Autodesk Fusion 360 part; units mm, degrees
(part 2 of 25)
  arc A218 (53.5347, 54.332) -> (53.2751, 54.0724) centre (53.5347, 54.0724) ccw
  arc A219 (53.5347, 54.3066) -> (53.5347, 54.3574) centre (53.5347, 54.332) ccw
  arc A220 (53.5996, 53.1763) -> (53.5996, 53.1255) centre (53.5996, 53.1509) ccw
  arc A221 (53.8988, 54.0724) -> (53.9496, 54.0724) centre (53.9242, 54.0724) ccw
  arc A222 (52.7304, 52.8264) -> (52.7812, 52.8264) centre (52.7558, 52.8264) ccw
  arc A223 (53.9242, 54.0724) -> (53.6646, 54.332) centre (53.6646, 54.0724) ccw
  arc A224 (53.8988, 53.6829) -> (53.9496, 53.6829) centre (53.9242, 53.6829) ccw
  arc A225 (52.7558, 53.7083) -> (52.7558, 53.6575) centre (52.7558, 53.6829) ccw
  arc A226 (34.8662, 27.9667) -> (34.8822, 28.0149) centre (34.8742, 27.9908) ccw
  arc A227 (53.2497, 53.6829) -> (53.3005, 53.6829) centre (53.2751, 53.6829) ccw
  arc A228 (53.3005, 54.0724) -> (53.2497, 54.0724) centre (53.2751, 54.0724) ccw
  arc A229 (53.0804, 53.1255) -> (53.0804, 53.1763) centre (53.0804, 53.1509) ccw
  arc A230 (53.2751, 53.6575) -> (53.2751, 53.7083) centre (53.2751, 53.6829) ccw
  arc A231 (52.7812, 54.332) -> (52.7304, 54.332) centre (52.7558, 54.332) ccw
  arc A232 (56.4642, 52.4764) -> (56.4642, 52.5272) centre (56.4642, 52.5018) ccw
  arc A233 (51.1246, 29.8986) -> (51.1246, 29.9494) centre (51.1246, 29.924) ccw
  line L54 (29.7942, 28.6399) -> (29.7942, 28.2504)
  arc A234 (52.7812, 52.8264) -> (52.7304, 52.8264) centre (52.7558, 52.8264) ccw
  arc A235 (53.8988, 52.5018) -> (53.9496, 52.5018) centre (53.9242, 52.5018) ccw
  line L55 (53.9242, 52.8264) -> (53.9242, 52.5018)
  arc A236 (53.2497, 54.0724) -> (53.3005, 54.0724) centre (53.2751, 54.0724) ccw
  arc A237 (54.9481, 2.4638) -> (54.9481, 2.5146) centre (54.9481, 2.4892) ccw
  arc A238 (55.3212, 52.8264) -> (55.2704, 52.8264) centre (55.2958, 52.8264) ccw
  arc A239 (53.0804, 53.1763) -> (53.0804, 53.1255) centre (53.0804, 53.1509) ccw
  arc A240 (55.2958, 52.5272) -> (55.2958, 52.4764) centre (55.2958, 52.5018) ccw
  arc A241 (53.6646, 54.3574) -> (53.6646, 54.3066) centre (53.6646, 54.332) ccw
  arc A242 (55.6204, 53.1509) -> (55.2958, 52.8264) centre (55.6204, 52.8263) ccw
  arc A243 (55.2704, 52.8264) -> (55.3212, 52.8264) centre (55.2958, 52.8264) ccw
  arc A244 (52.7304, 52.5018) -> (52.7812, 52.5018) centre (52.7558, 52.5018) ccw
  arc A245 (53.8988, 52.8264) -> (53.9496, 52.8264) centre (53.9242, 52.8264) ccw
  arc A246 (53.9496, 54.0724) -> (53.8988, 54.0724) centre (53.9242, 54.0724) ccw
  line L56 (52.7558, 53.6829) -> (52.7558, 54.332)
  arc A247 (52.7304, 53.6829) -> (52.7812, 53.6829) centre (52.7558, 53.6829) ccw
  arc A248 (52.7558, 52.5272) -> (52.7558, 52.4764) centre (52.7558, 52.5018) ccw
  arc A249 (28.8854, 28.0162) -> (28.8854, 27.9654) centre (28.8854, 27.9908) ccw
  arc A250 (26.0778, 30.3771) -> (26.0938, 30.3289) centre (26.0858, 30.353) ccw
  line L57 (53.0804, 53.1509) -> (53.5996, 53.1509)
  arc A251 (26.0604, 29.2749) -> (26.1112, 29.2749) centre (26.0858, 29.2749) ccw
  arc A252 (33.7138, 28.4044) -> (33.6978, 28.3562) centre (33.7058, 28.3803) ccw
  arc A253 (53.9242, 52.8264) -> (53.5996, 53.1509) centre (53.5996, 52.8263) ccw
  line L58 (53.9242, 53.6829) -> (53.9242, 54.0724)
  line L59 (53.2751, 54.0724) -> (53.2751, 53.6829)
  arc A254 (29.8196, 28.6399) -> (29.7688, 28.6399) centre (29.7942, 28.6399) ccw
  line L60 (53.2751, 53.6829) -> (52.7558, 53.6829)
  line L61 (55.6204, 53.1509) -> (56.1396, 53.1509)
  line L62 (55.2958, 52.5018) -> (55.2958, 52.8264)
  arc A255 (56.1396, 53.1255) -> (56.1396, 53.1763) centre (56.1396, 53.1509) ccw
  arc A256 (61.5442, 52.8264) -> (61.2196, 53.1509) centre (61.2196, 52.8263) ccw
  arc A257 (56.23, 54.332) -> (56.1792, 54.332) centre (56.2046, 54.332) ccw
  arc A258 (58.1604, 53.1763) -> (58.1604, 53.1255) centre (58.1604, 53.1509) ccw
  line L63 (59.0042, 53.6829) -> (59.0042, 54.0075)
  arc A259 (59.0042, 54.0075) -> (58.3551, 54.0075) centre (58.6797, 54.0075) ccw
  arc A260 (55.3028, 53.967) -> (55.2888, 53.9181) centre (55.2958, 53.9426) ccw
  arc A261 (58.1604, 53.1509) -> (57.8358, 52.8264) centre (58.1604, 52.8263) ccw
  line L64 (56.2046, 53.6829) -> (56.2046, 54.332)
  arc A262 (58.3297, 54.0075) -> (58.3805, 54.0075) centre (58.3551, 54.0075) ccw
  arc A263 (57.8612, 52.8264) -> (57.8104, 52.8264) centre (57.8358, 52.8264) ccw
  arc A264 (57.8104, 53.6829) -> (57.8612, 53.6829) centre (57.8358, 53.6829) ccw
  arc A265 (56.1792, 53.6829) -> (56.23, 53.6829) centre (56.2046, 53.6829) ccw
  arc A266 (58.1604, 53.1255) -> (58.1604, 53.1763) centre (58.1604, 53.1509) ccw
  arc A267 (58.3551, 54.0724) -> (57.8358, 54.0724) centre (58.0954, 54.0724) ccw
  arc A268 (56.4896, 52.8264) -> (56.4388, 52.8264) centre (56.4642, 52.8264) ccw
  arc A269 (58.3297, 54.0724) -> (58.3805, 54.0724) centre (58.3551, 54.0724) ccw
  arc A270 (59.0296, 52.8264) -> (58.9788, 52.8264) centre (59.0042, 52.8264) ccw
  arc A271 (60.3758, 52.5272) -> (60.3758, 52.4764) centre (60.3758, 52.5018) ccw
  arc A272 (61.5442, 52.4764) -> (61.5442, 52.5272) centre (61.5442, 52.5018) ccw
  line L65 (61.5442, 52.5018) -> (60.3758, 52.5018)
  arc A273 (58.3297, 53.8127) -> (58.3805, 53.8127) centre (58.3551, 53.8127) ccw
  arc A274 (60.4012, 52.8264) -> (60.3504, 52.8264) centre (60.3758, 52.8264) ccw
  line L66 (59.0042, 52.5018) -> (57.8358, 52.5018)
  line L67 (55.9449, 54.1373) -> (56.4642, 54.1373)
  line L68 (59.0042, 52.8264) -> (59.0042, 52.5018)
  arc A275 (58.9788, 53.6829) -> (59.0296, 53.6829) centre (59.0042, 53.6829) ccw
  arc A276 (60.7004, 53.1509) -> (60.3758, 52.8264) centre (60.7004, 52.8263) ccw
  arc A277 (57.8104, 52.5018) -> (57.8612, 52.5018) centre (57.8358, 52.5018) ccw
  line L69 (60.7004, 53.1509) -> (61.2196, 53.1509)
  arc A278 (59.0042, 52.8264) -> (58.6796, 53.1509) centre (58.6796, 52.8263) ccw
  arc A279 (58.9788, 52.8264) -> (59.0296, 52.8264) centre (59.0042, 52.8264) ccw
  arc A280 (60.3504, 52.8264) -> (60.4012, 52.8264) centre (60.3758, 52.8264) ccw
  arc A281 (57.8612, 54.0724) -> (57.8104, 54.0724) centre (57.8358, 54.0724) ccw
  arc A282 (60.7004, 53.1763) -> (60.7004, 53.1255) centre (60.7004, 53.1509) ccw
  arc A283 (55.9449, 54.1627) -> (55.9449, 54.1119) centre (55.9449, 54.1373) ccw
  line L70 (57.8358, 52.5018) -> (57.8358, 52.8264)
  arc A284 (57.8104, 52.8264) -> (57.8612, 52.8264) centre (57.8358, 52.8264) ccw
  arc A285 (60.7004, 53.1255) -> (60.7004, 53.1763) centre (60.7004, 53.1509) ccw
  line L71 (58.3551, 54.0724) -> (58.3551, 53.8127)
  arc A286 (55.6204, 53.1763) -> (55.6204, 53.1255) centre (55.6204, 53.1509) ccw
  arc A287 (57.8358, 52.5272) -> (57.8358, 52.4764) centre (57.8358, 52.5018) ccw
  arc A288 (59.0042, 52.4764) -> (59.0042, 52.5272) centre (59.0042, 52.5018) ccw
  arc A289 (56.4642, 52.8264) -> (56.1396, 53.1509) centre (56.1396, 52.8263) ccw
  arc A290 (58.9788, 54.0075) -> (59.0296, 54.0075) centre (59.0042, 54.0075) ccw
  arc A291 (56.4388, 52.5018) -> (56.4896, 52.5018) centre (56.4642, 52.5018) ccw
  line L72 (56.4642, 52.8264) -> (56.4642, 52.5018)
  arc A292 (56.1976, 53.6585) -> (56.2115, 53.7073) centre (56.2045, 53.6829) ccw
  arc A293 (56.4642, 54.1119) -> (56.4642, 54.1627) centre (56.4642, 54.1373) ccw
  arc A294 (58.6796, 53.1255) -> (58.6796, 53.1763) centre (58.6796, 53.1509) ccw
  arc A295 (58.6796, 53.1763) -> (58.6796, 53.1255) centre (58.6796, 53.1509) ccw
  arc A296 (59.0296, 54.0075) -> (58.9788, 54.0075) centre (59.0042, 54.0075) ccw
  line L73 (58.1604, 53.1509) -> (58.6796, 53.1509)
  arc A297 (58.9788, 52.5018) -> (59.0296, 52.5018) centre (59.0042, 52.5018) ccw
  line L74 (55.2958, 53.9425) -> (56.2046, 53.6829)
  arc A298 (58.3805, 54.0724) -> (58.3297, 54.0724) centre (58.3551, 54.0724) ccw
  line L75 (57.8358, 53.6829) -> (57.8358, 54.0724)
  arc A299 (56.1396, 53.1763) -> (56.1396, 53.1255) centre (56.1396, 53.1509) ccw
  line L76 (60.3758, 52.5018) -> (60.3758, 52.8264)
  arc A300 (57.8104, 54.0724) -> (57.8612, 54.0724) centre (57.8358, 54.0724) ccw
  arc A301 (60.3504, 52.5018) -> (60.4012, 52.5018) centre (60.3758, 52.5018) ccw
  arc A302 (61.2196, 53.1255) -> (61.2196, 53.1763) centre (61.2196, 53.1509) ccw
  arc A303 (31.1578, 28.4044) -> (31.1738, 28.3562) centre (31.1658, 28.3803) ccw
  arc A304 (32.3422, 28.7456) -> (32.3262, 28.7938) centre (32.3342, 28.7697) ccw
  arc A305 (32.3262, 27.9667) -> (32.3422, 28.0149) centre (32.3342, 27.9908) ccw
  arc A306 (31.1738, 28.4044) -> (31.1578, 28.3562) centre (31.1658, 28.3803) ccw
  line L77 (31.4254, 29.1987) -> (31.1658, 29.5233)
  line L78 (61.5442, 53.6829) -> (61.5442, 54.332)
  line L79 (58.1604, 9.5899) -> (58.6796, 9.5899)
  arc A307 (60.6679, 54.3066) -> (60.6679, 54.3574) centre (60.6679, 54.332) ccw
  arc A308 (61.2196, 53.1763) -> (61.2196, 53.1255) centre (61.2196, 53.1509) ccw
  arc A309 (60.6276, 53.6587) -> (60.6433, 53.7071) centre (60.6355, 53.6829) ccw
  arc A310 (60.8951, 54.2346) -> (60.6679, 54.332) centre (60.6679, 54.0183) ccw
  line L80 (57.8358, 8.9408) -> (57.8358, 9.2654)
  arc A311 (61.5188, 52.5018) -> (61.5696, 52.5018) centre (61.5442, 52.5018) ccw
  arc A312 (60.6679, 54.332) -> (60.3758, 54.0399) centre (60.6679, 54.0399) ccw
  arc A313 (61.5696, 54.332) -> (61.5188, 54.332) centre (61.5442, 54.332) ccw
  line L81 (57.8358, 10.4465) -> (59.0042, 10.4465)
  line L82 (28.6258, 28.2504) -> (28.6258, 28.6399)
  arc A314 (57.8358, 8.9662) -> (57.8358, 8.9154) centre (57.8358, 8.9408) ccw
  line L83 (59.0042, 8.9408) -> (57.8358, 8.9408)
  arc A315 (57.8556, 10.4623) -> (57.816, 10.4306) centre (57.8358, 10.4465) ccw
  line L84 (59.0042, 10.1219) -> (59.0042, 10.771)
  arc A316 (32.3342, 29.4979) -> (32.3342, 29.5487) centre (32.3342, 29.5233) ccw
  arc A317 (60.4012, 54.0399) -> (60.3504, 54.0399) centre (60.3758, 54.0399) ccw
  arc A318 (60.6679, 54.3574) -> (60.6679, 54.3066) centre (60.6679, 54.332) ccw
  arc A319 (58.9788, 8.9408) -> (59.0296, 8.9408) centre (59.0042, 8.9408) ccw
  arc A320 (58.9788, 9.2654) -> (59.0296, 9.2654) centre (59.0042, 9.2654) ccw
  line L85 (61.5442, 52.8264) -> (61.5442, 52.5018)
  arc A321 (61.5696, 52.8264) -> (61.5188, 52.8264) centre (61.5442, 52.8264) ccw
  arc A322 (32.0167, 28.0882) -> (32.0675, 28.0882) centre (32.0421, 28.0882) ccw
  line L86 (32.3342, 29.1987) -> (32.3342, 29.8478)
  arc A323 (59.0042, 8.9154) -> (59.0042, 8.9662) centre (59.0042, 8.9408) ccw
  arc A324 (57.8358, 10.4718) -> (57.8358, 10.4211) centre (57.8358, 10.4465) ccw
  arc A325 (31.1658, 29.5487) -> (31.1658, 29.4979) centre (31.1658, 29.5233) ccw
  arc A326 (61.5188, 53.6829) -> (61.5696, 53.6829) centre (61.5442, 53.6829) ccw
  arc A327 (57.8612, 9.2654) -> (57.8104, 9.2654) centre (57.8358, 9.2654) ccw
  arc A328 (60.3758, 54.0399) -> (60.6354, 53.6829) centre (60.751, 54.0399) ccw
  arc A329 (61.5277, 53.6635) -> (61.5607, 53.7023) centre (61.5442, 53.6829) ccw
  line L87 (58.0954, 10.1219) -> (57.8358, 10.4465)
  arc A330 (59.0296, 9.2654) -> (58.9788, 9.2654) centre (59.0042, 9.2654) ccw
  arc A331 (58.1604, 9.5899) -> (57.8358, 9.2654) centre (58.1604, 9.2653) ccw
  arc A332 (60.3504, 54.0399) -> (60.4012, 54.0399) centre (60.3758, 54.0399) ccw
  arc A333 (58.6796, 9.5645) -> (58.6796, 9.6153) centre (58.6796, 9.5899) ccw
  arc A334 (59.0042, 10.4211) -> (59.0042, 10.4718) centre (59.0042, 10.4465) ccw
  arc A335 (61.5188, 52.8264) -> (61.5696, 52.8264) centre (61.5442, 52.8264) ccw
  arc A336 (60.9115, 54.254) -> (60.8786, 54.2153) centre (60.895, 54.2347) ccw
  line L88 (59.0042, 9.2654) -> (59.0042, 8.9408)
  arc A337 (31.4056, 29.1828) -> (31.4453, 29.2146) centre (31.4255, 29.1987) ccw
  arc A338 (31.1856, 29.5391) -> (31.146, 29.5074) centre (31.1658, 29.5233) ccw
  line L89 (34.8742, 27.9908) -> (33.7058, 28.3803)
  line L90 (31.1658, 29.5233) -> (32.3342, 29.5233)
  arc A339 (60.8767, 54.2171) -> (60.9135, 54.2522) centre (60.8951, 54.2346) ccw
  arc A340 (57.8104, 8.9408) -> (57.8612, 8.9408) centre (57.8358, 8.9408) ccw
  arc A341 (32.3088, 29.1987) -> (32.3596, 29.1987) centre (32.3342, 29.1987) ccw
  arc A342 (57.8104, 9.2654) -> (57.8612, 9.2654) centre (57.8358, 9.2654) ccw
  line L91 (34.5821, 28.6724) -> (34.5821, 28.0882)
  arc A343 (59.0042, 9.2654) -> (58.6796, 9.5899) centre (58.6796, 9.2653) ccw
  arc A344 (58.1604, 9.5645) -> (58.1604, 9.6153) centre (58.1604, 9.5899) ccw
  arc A345 (58.0756, 10.106) -> (58.1153, 10.1378) centre (58.0954, 10.1219) ccw
  line L92 (60.8951, 54.2346) -> (61.5442, 53.6829)
  arc A346 (32.3596, 29.8478) -> (32.3088, 29.8478) centre (32.3342, 29.8478) ccw
  arc A347 (58.6796, 9.6153) -> (58.6796, 9.5645) centre (58.6796, 9.5899) ccw
  line L93 (33.7058, 28.3803) -> (34.8742, 28.7697)
  arc A348 (58.1604, 9.6153) -> (58.1604, 9.5645) centre (58.1604, 9.5899) ccw
  arc A349 (32.0675, 28.6724) -> (32.0167, 28.6724) centre (32.0421, 28.6724) ccw
  arc A350 (28.6258, 29.2354) -> (28.6258, 29.1846) centre (28.6258, 29.21) ccw
  line L94 (70.485, 34.29) -> (52.07, 34.29)
  arc A351 (51.9938, 34.29) -> (52.1462, 34.29) centre (52.07, 34.29) ccw
  arc A352 (29.1705, 28.6399) -> (29.1197, 28.6399) centre (29.1451, 28.6399) ccw
  arc A353 (29.8065, 29.8369) -> (29.7819, 29.8813) centre (29.7942, 29.8591) ccw
  arc A354 (26.9946, 29.8986) -> (26.9946, 29.9494) centre (26.9946, 29.924) ccw
  arc A355 (29.7942, 52.6429) -> (29.7434, 52.6429) centre (29.7688, 52.6429) ccw
  arc A356 (29.7942, 30.4038) -> (29.7942, 30.4546) centre (29.7942, 30.4292) ccw
  arc A357 (29.7688, 52.2534) -> (30.0284, 51.9938) centre (30.0284, 52.2534) ccw
  arc A358 (28.9504, 31.0783) -> (28.6258, 30.7537) centre (28.9504, 30.7537) ccw
  line L95 (26.0858, 29.2749) -> (26.0858, 29.924)
  arc A359 (52.07, 40.7162) -> (52.07, 40.5638) centre (52.07, 40.64) ccw
  arc A360 (70.4088, 34.29) -> (70.5612, 34.29) centre (70.485, 34.29) ccw
  arc A361 (52.1462, 40.64) -> (51.9938, 40.64) centre (52.07, 40.64) ccw
  arc A362 (29.7942, 30.7537) -> (29.4696, 31.0783) centre (29.4696, 30.7537) ccw
  arc A363 (28.6004, 30.7537) -> (28.6512, 30.7537) centre (28.6258, 30.7537) ccw
  arc A364 (28.9504, 31.0529) -> (28.9504, 31.1037) centre (28.9504, 31.0783) ccw
  line L96 (31.1658, 28.3803) -> (32.3342, 28.7697)
  arc A365 (28.6512, 28.2504) -> (28.6004, 28.2504) centre (28.6258, 28.2504) ccw
  arc A366 (70.485, 40.5638) -> (70.485, 40.7162) centre (70.485, 40.64) ccw
  line L97 (29.7688, 52.2534) -> (29.7688, 52.6429)
  arc A367 (29.7942, 52.2534) -> (29.7434, 52.2534) centre (29.7688, 52.2534) ccw
  arc A368 (28.6135, 29.2322) -> (28.6381, 29.1878) centre (28.6258, 29.21) ccw
  arc A369 (28.6258, 30.4546) -> (28.6258, 30.4038) centre (28.6258, 30.4292) ccw
  line L98 (28.6258, 30.4292) -> (28.6258, 30.7537)
  arc A370 (28.9504, 31.1037) -> (28.9504, 31.0529) centre (28.9504, 31.0783) ccw
  arc A371 (70.485, 34.2138) -> (70.485, 34.3662) centre (70.485, 34.29) ccw
  line L99 (29.7688, 53.213) -> (30.9372, 53.8621)
  arc A372 (50.9947, 29.9494) -> (50.9947, 29.8986) centre (50.9947, 29.924) ccw
  arc A373 (28.6512, 30.7537) -> (28.6004, 30.7537) centre (28.6258, 30.7537) ccw
  arc A374 (29.4696, 31.1037) -> (29.4696, 31.0529) centre (29.4696, 31.0783) ccw
  arc A375 (29.7688, 53.2384) -> (29.7688, 53.1876) centre (29.7688, 53.213) ccw
  arc A376 (52.07, 34.3662) -> (52.07, 34.2138) centre (52.07, 34.29) ccw
  arc A377 (29.7688, 30.4292) -> (29.8196, 30.4292) centre (29.7942, 30.4292) ccw
  arc A378 (29.8196, 30.7537) -> (29.7688, 30.7537) centre (29.7942, 30.7537) ccw
  line L100 (52.07, 40.64) -> (70.485, 40.64)
  line L101 (33.6042, 52.5018) -> (32.4358, 52.5018)
  arc A379 (28.8854, 27.9654) -> (28.8854, 28.0162) centre (28.8854, 27.9908) ccw
  arc A380 (28.6004, 30.4292) -> (28.6512, 30.4292) centre (28.6258, 30.4292) ccw
  line L102 (29.7942, 30.4292) -> (28.6258, 30.4292)
  arc A381 (29.7688, 30.7537) -> (29.8196, 30.7537) centre (29.7942, 30.7537) ccw
  line L103 (32.3342, 27.9908) -> (31.1658, 28.3803)
  arc A382 (29.5346, 27.9654) -> (29.5346, 28.0162) centre (29.5346, 27.9908) ccw
  line L104 (52.07, 34.29) -> (52.07, 40.64)
  line L105 (32.0421, 28.6724) -> (32.0421, 28.0882)
  arc A383 (30.0284, 51.9684) -> (30.0284, 52.0192) centre (30.0284, 51.9938) ccw
  arc A384 (28.6258, 29.8845) -> (28.6258, 29.8337) centre (28.6258, 29.8591) ccw
  arc A385 (29.7434, 52.2534) -> (29.7942, 52.2534) centre (29.7688, 52.2534) ccw
  arc A386 (29.7942, 29.8337) -> (29.7942, 29.8845) centre (29.7942, 29.8591) ccw
  arc A387 (54.6885, 2.5146) -> (54.6885, 2.4638) centre (54.6885, 2.4892) ccw
  arc A388 (54.9481, 1.2954) -> (54.9481, 1.3462) centre (54.9481, 1.3208) ccw
  arc A389 (51.1246, 29.9494) -> (51.1246, 29.8986) centre (51.1246, 29.924) ccw
  line L106 (70.485, 40.64) -> (70.485, 34.29)
  arc A390 (29.7942, 29.1846) -> (29.7942, 29.2354) centre (29.7942, 29.21) ccw
  arc A391 (28.6258, 28.2504) -> (28.8854, 27.9908) centre (28.8854, 28.2504) ccw
  arc A392 (70.5612, 40.64) -> (70.4088, 40.64) centre (70.485, 40.64) ccw
  arc A393 (28.6004, 28.2504) -> (28.6512, 28.2504) centre (28.6258, 28.2504) ccw
  line L107 (29.7942, 30.7537) -> (29.7942, 30.4292)
  arc A394 (28.6512, 28.6399) -> (28.6004, 28.6399) centre (28.6258, 28.6399) ccw
  line L108 (29.7942, 29.8591) -> (28.6258, 29.8591)
  arc A395 (54.4542, 2.2296) -> (54.4034, 2.2296) centre (54.4288, 2.2296) ccw
  arc A396 (54.4288, 1.5804) -> (54.6885, 1.3208) centre (54.6885, 1.5805) ccw
  line L109 (29.7942, 29.21) -> (28.6258, 29.21)
  arc A397 (29.4696, 31.0529) -> (29.4696, 31.1037) centre (29.4696, 31.0783) ccw
  arc A398 (40.9646, 8.9662) -> (40.9646, 8.9154) centre (40.9646, 8.9408) ccw
  arc A399 (26.0096, 53.9355) -> (25.9588, 53.9355) centre (25.9842, 53.9355) ccw
  line L110 (25.9842, 52.8913) -> (24.8158, 53.2807)
  arc A400 (25.9842, 53.7803) -> (25.9842, 53.8311) centre (25.9842, 53.8057) ccw
  arc A401 (24.8412, 53.9355) -> (24.7904, 53.9355) centre (24.8158, 53.9355) ccw
  arc A402 (30.9372, 54.7567) -> (30.6126, 55.0813) centre (30.6126, 54.7567) ccw
  arc A403 (30.9372, 53.8367) -> (30.9372, 53.8875) centre (30.9372, 53.8621) ccw
  line L111 (28.6258, 29.21) -> (29.7942, 29.8591)
  arc A404 (25.9842, 54.4082) -> (25.9842, 54.459) centre (25.9842, 54.4336) ccw
  arc A405 (30.9372, 53.1876) -> (30.9372, 53.2384) centre (30.9372, 53.213) ccw
  arc A406 (30.0934, 55.1067) -> (30.0934, 55.0559) centre (30.0934, 55.0813) ccw
  line L112 (24.8158, 54.4336) -> (25.9842, 55.0827)
  arc A407 (30.9118, 54.4322) -> (30.9626, 54.4322) centre (30.9372, 54.4322) ccw
  line L113 (40.0558, 11.3792) -> (40.0558, 11.7037)
  arc A408 (26.5797, 29.2749) -> (26.6305, 29.2749) centre (26.6051, 29.2749) ccw
  line L114 (41.2242, 10.16) -> (40.0558, 10.16)
  line L115 (40.9646, 8.9408) -> (40.3154, 8.9408)
  arc A409 (40.3154, 8.9662) -> (40.3154, 8.9154) centre (40.3154, 8.9408) ccw
  line L116 (24.8158, 53.8057) -> (25.9842, 53.8057)
  line L117 (40.5751, 9.3952) -> (40.5751, 9.5899)
  line L118 (41.2242, 9.5899) -> (41.2242, 9.2004)
  arc A410 (40.0812, 9.5899) -> (40.0304, 9.5899) centre (40.0558, 9.5899) ccw
  arc A411 (40.9646, 8.9154) -> (40.9646, 8.9662) centre (40.9646, 8.9408) ccw
  arc A412 (40.3154, 8.9154) -> (40.3154, 8.9662) centre (40.3154, 8.9408) ccw
  line L119 (30.9372, 53.213) -> (29.7688, 53.213)
  line L120 (30.9372, 54.4322) -> (29.7688, 54.4322)
  arc A413 (30.9372, 54.4068) -> (30.9372, 54.4576) centre (30.9372, 54.4322) ccw
  arc A414 (29.7942, 54.7567) -> (29.7434, 54.7567) centre (29.7688, 54.7567) ccw
  line L121 (25.9842, 53.6758) -> (25.9842, 53.9355)
  line L122 (30.9372, 54.7567) -> (30.9372, 54.4322)
  arc A415 (25.9762, 52.8672) -> (25.9922, 52.9154) centre (25.9842, 52.8913) ccw
  arc A416 (24.8238, 53.3048) -> (24.8078, 53.2566) centre (24.8158, 53.2807) ccw
  arc A417 (30.9626, 54.7567) -> (30.9118, 54.7567) centre (30.9372, 54.7567) ccw
  arc A418 (40.5751, 9.6153) -> (40.5751, 9.5645) centre (40.5751, 9.5899) ccw
  arc A419 (24.7904, 53.6758) -> (24.8412, 53.6758) centre (24.8158, 53.6758) ccw
  line L123 (40.0558, 10.16) -> (41.2242, 10.8091)
  line L124 (30.9372, 53.8621) -> (29.7688, 53.8621)
  arc A420 (29.7434, 54.7567) -> (29.7942, 54.7567) centre (29.7688, 54.7567) ccw
  arc A421 (30.6126, 55.0559) -> (30.6126, 55.1067) centre (30.6126, 55.0813) ccw
  arc A422 (29.7688, 53.8875) -> (29.7688, 53.8367) centre (29.7688, 53.8621) ccw
  arc A423 (30.6126, 55.1067) -> (30.6126, 55.0559) centre (30.6126, 55.0813) ccw
  arc A424 (24.8158, 54.459) -> (24.8158, 54.4082) centre (24.8158, 54.4336) ccw
  arc A425 (30.9118, 54.7567) -> (30.9626, 54.7567) centre (30.9372, 54.7567) ccw
  arc A426 (30.0934, 55.0813) -> (29.7688, 54.7567) centre (30.0934, 54.7567) ccw
  arc A427 (29.7434, 54.4322) -> (29.7942, 54.4322) centre (29.7688, 54.4322) ccw
  line L125 (24.8158, 53.6758) -> (24.8158, 53.9355)
  line L126 (24.8158, 52.5018) -> (25.9842, 52.8913)
  arc A428 (40.0812, 9.2004) -> (40.0304, 9.2004) centre (40.0558, 9.2004) ccw
  arc A429 (25.9922, 52.8672) -> (25.9762, 52.9154) centre (25.9842, 52.8913) ccw
  line L127 (40.0558, 9.2004) -> (40.0558, 9.5899)
  arc A430 (24.8078, 52.5259) -> (24.8238, 52.4777) centre (24.8158, 52.5018) ccw
  arc A431 (24.8158, 53.8311) -> (24.8158, 53.7803) centre (24.8158, 53.8057) ccw
  arc A432 (29.8196, 28.2504) -> (29.7688, 28.2504) centre (29.7942, 28.2504) ccw
  arc A433 (30.9495, 53.8399) -> (30.9249, 53.8843) centre (30.9372, 53.8621) ccw
  line L128 (30.0934, 55.0813) -> (30.6126, 55.0813)
  line L129 (29.7688, 54.4322) -> (29.7688, 54.7567)
  arc A434 (30.0934, 55.0559) -> (30.0934, 55.1067) centre (30.0934, 55.0813) ccw
  arc A435 (41.1988, 9.2004) -> (41.2496, 9.2004) centre (41.2242, 9.2004) ccw
  arc A436 (25.9588, 53.6758) -> (26.0096, 53.6758) centre (25.9842, 53.6758) ccw
  arc A437 (40.0558, 10.8345) -> (40.0558, 10.7837) centre (40.0558, 10.8091) ccw
  arc A438 (29.7688, 54.4576) -> (29.7688, 54.4068) centre (29.7688, 54.4322) ccw
  line L130 (25.9842, 54.4336) -> (24.8158, 54.4336)
  arc A439 (29.7565, 53.2352) -> (29.7811, 53.1908) centre (29.7688, 53.213) ccw
  arc A440 (27.2622, 30.7184) -> (27.2462, 30.7666) centre (27.2542, 30.7425) ccw
  arc A441 (37.1475, 28.6724) -> (37.0967, 28.6724) centre (37.1221, 28.6724) ccw
  arc A442 (40.9646, 8.9408) -> (41.2242, 9.2004) centre (40.9646, 9.2004) ccw
  arc A443 (40.8996, 12.0029) -> (40.8996, 12.0537) centre (40.8996, 12.0283) ccw
  arc A444 (40.8996, 12.0537) -> (40.8996, 12.0029) centre (40.8996, 12.0283) ccw
  arc A445 (40.0558, 11.4046) -> (40.0558, 11.3538) centre (40.0558, 11.3792) ccw
  arc A446 (40.0304, 9.2004) -> (40.0812, 9.2004) centre (40.0558, 9.2004) ccw
  arc A447 (40.3804, 12.0283) -> (40.0558, 11.7037) centre (40.3804, 11.7037) ccw
  arc A448 (41.2365, 10.7869) -> (41.2119, 10.8313) centre (41.2242, 10.8091) ccw
  arc A449 (40.6005, 9.5899) -> (40.5497, 9.5899) centre (40.5751, 9.5899) ccw
  arc A450 (40.0435, 10.1822) -> (40.0681, 10.1378) centre (40.0558, 10.16) ccw
  arc A451 (40.0304, 11.3792) -> (40.0812, 11.3792) centre (40.0558, 11.3792) ccw
  arc A452 (41.2242, 11.7037) -> (40.8996, 12.0283) centre (40.8996, 11.7037) ccw
  arc A453 (41.2242, 11.3538) -> (41.2242, 11.4046) centre (41.2242, 11.3792) ccw
  arc A454 (40.0558, 10.1854) -> (40.0558, 10.1346) centre (40.0558, 10.16) ccw
  arc A455 (41.1988, 11.7037) -> (41.2496, 11.7037) centre (41.2242, 11.7037) ccw
  line L131 (30.2881, 52.6429) -> (30.9372, 52.6429)
  line L132 (41.2242, 11.7037) -> (41.2242, 11.3792)
  arc A456 (30.2881, 52.6683) -> (30.2881, 52.6175) centre (30.2881, 52.6429) ccw
  arc A457 (41.2242, 10.1346) -> (41.2242, 10.1854) centre (41.2242, 10.16) ccw
  arc A458 (30.9118, 52.2534) -> (30.9626, 52.2534) centre (30.9372, 52.2534) ccw
  line L133 (30.6776, 51.9938) -> (30.0284, 51.9938)
  arc A459 (41.2496, 11.7037) -> (41.1988, 11.7037) centre (41.2242, 11.7037) ccw
  arc A460 (41.2242, 9.5645) -> (41.2242, 9.6153) centre (41.2242, 9.5899) ccw
  arc A461 (40.0812, 11.7037) -> (40.0304, 11.7037) centre (40.0558, 11.7037) ccw
  arc A462 (30.9626, 52.6429) -> (30.9118, 52.6429) centre (30.9372, 52.6429) ccw
  arc A463 (41.2242, 10.7837) -> (41.2242, 10.8345) centre (41.2242, 10.8091) ccw
  line L134 (30.2881, 52.4482) -> (30.2881, 52.6429)
  arc A464 (30.6776, 51.9938) -> (30.9372, 52.2534) centre (30.6776, 52.2534) ccw
  arc A465 (30.6776, 52.0192) -> (30.6776, 51.9684) centre (30.6776, 51.9938) ccw
  arc A466 (30.0284, 52.0192) -> (30.0284, 51.9684) centre (30.0284, 51.9938) ccw
  arc A467 (30.6776, 51.9684) -> (30.6776, 52.0192) centre (30.6776, 51.9938) ccw
  line L135 (36.0299, 1.3208) -> (36.679, 1.3208)
  arc A468 (36.329, 1.3208) -> (36.3798, 1.3208) centre (36.3544, 1.3208) ccw
  line L136 (41.2242, 10.8091) -> (40.0558, 10.8091)
  arc A469 (40.3804, 12.0537) -> (40.3804, 12.0029) centre (40.3804, 12.0283) ccw
  arc A470 (40.5497, 9.3952) -> (40.6005, 9.3952) centre (40.5751, 9.3952) ccw
  arc A471 (38.7096, 11.7037) -> (38.6588, 11.7037) centre (38.6842, 11.7037) ccw
  arc A472 (30.3135, 52.6429) -> (30.2627, 52.6429) centre (30.2881, 52.6429) ccw
  arc A473 (34.2415, 29.7698) -> (34.2086, 29.7311) centre (34.2251, 29.7505) ccw
  arc A474 (30.2627, 52.4482) -> (30.3135, 52.4482) centre (30.2881, 52.4482) ccw
  arc A475 (41.2496, 9.2004) -> (41.1988, 9.2004) centre (41.2242, 9.2004) ccw
  line L137 (40.3804, 12.0283) -> (40.8996, 12.0283)
  arc A476 (30.9372, 52.6175) -> (30.9372, 52.6683) centre (30.9372, 52.6429) ccw
  line L138 (30.9372, 52.6429) -> (30.9372, 52.2534)
  arc A477 (41.2496, 9.5899) -> (41.1988, 9.5899) centre (41.2242, 9.5899) ccw
  line L139 (41.2242, 11.3792) -> (40.0558, 11.3792)
  arc A478 (30.9626, 52.2534) -> (30.9118, 52.2534) centre (30.9372, 52.2534) ccw
  arc A479 (34.8488, 29.1987) -> (34.8996, 29.1987) centre (34.8742, 29.1987) ccw
  arc A480 (34.8996, 29.8478) -> (34.8488, 29.8478) centre (34.8742, 29.8478) ccw
  line L140 (37.4142, 27.9908) -> (36.2458, 28.3803)
  line L141 (40.5751, 9.5899) -> (41.2242, 9.5899)
  arc A481 (36.2378, 28.4044) -> (36.2538, 28.3562) centre (36.2458, 28.3803) ccw
  arc A482 (41.1988, 11.3792) -> (41.2496, 11.3792) centre (41.2242, 11.3792) ccw
  line L142 (36.2458, 28.3803) -> (37.4142, 28.7697)
  line L143 (34.8742, 29.1987) -> (34.8742, 29.8478)
  line L144 (51.1246, 29.924) -> (50.9947, 29.924)
  arc A483 (37.4062, 27.9667) -> (37.4222, 28.0149) centre (37.4142, 27.9908) ccw
  arc A484 (37.4222, 28.7456) -> (37.4062, 28.7938) centre (37.4142, 28.7697) ccw
  arc A485 (40.0558, 9.2004) -> (40.3154, 8.9408) centre (40.3154, 9.2004) ccw
  arc A486 (40.3804, 12.0029) -> (40.3804, 12.0537) centre (40.3804, 12.0283) ccw
  arc A487 (36.2538, 28.4044) -> (36.2378, 28.3562) centre (36.2458, 28.3803) ccw
  arc A488 (40.0304, 11.7037) -> (40.0812, 11.7037) centre (40.0558, 11.7037) ccw
  line L145 (37.1221, 28.6724) -> (37.1221, 28.0882)
  arc A489 (37.3888, 29.1987) -> (37.4396, 29.1987) centre (37.4142, 29.1987) ccw
  arc A490 (53.9242, 30.4038) -> (53.9242, 30.4546) centre (53.9242, 30.4292) ccw
  arc A491 (53.0804, 31.0529) -> (53.0804, 31.1037) centre (53.0804, 31.0783) ccw
  arc A492 (53.3005, 28.6399) -> (53.2497, 28.6399) centre (53.2751, 28.6399) ccw
  arc A493 (52.7435, 29.2322) -> (52.7681, 29.1878) centre (52.7558, 29.21) ccw
  arc A494 (53.8988, 30.4292) -> (53.9496, 30.4292) centre (53.9242, 30.4292) ccw
  arc A495 (52.7304, 30.7537) -> (52.7812, 30.7537) centre (52.7558, 30.7537) ccw
  arc A496 (36.7397, 29.3285) -> (36.7905, 29.3285) centre (36.7651, 29.3285) ccw
  line L146 (36.2458, 29.1987) -> (36.2458, 29.5882)
  arc A497 (52.7304, 28.2504) -> (52.7812, 28.2504) centre (52.7558, 28.2504) ccw
  arc A498 (53.0154, 28.0162) -> (53.0154, 27.9654) centre (53.0154, 27.9908) ccw
  arc A499 (53.8988, 30.7537) -> (53.9496, 30.7537) centre (53.9242, 30.7537) ccw
  arc A500 (37.3888, 29.5233) -> (37.4396, 29.5233) centre (37.4142, 29.5233) ccw
  arc A501 (53.9242, 30.7537) -> (53.5996, 31.0783) centre (53.5996, 30.7537) ccw
  arc A502 (53.5996, 31.0529) -> (53.5996, 31.1037) centre (53.5996, 31.0783) ccw
  arc A503 (52.7558, 28.2504) -> (53.0154, 27.9908) centre (53.0154, 28.2504) ccw
  arc A504 (53.0154, 27.9654) -> (53.0154, 28.0162) centre (53.0154, 27.9908) ccw
  arc A505 (52.7558, 29.2354) -> (52.7558, 29.1846) centre (52.7558, 29.21) ccw
  arc A506 (37.4396, 29.5233) -> (37.3888, 29.5233) centre (37.4142, 29.5233) ccw
  arc A507 (53.0804, 31.0783) -> (52.7558, 30.7537) centre (53.0804, 30.7537) ccw
  arc A508 (53.0804, 31.1037) -> (53.0804, 31.0529) centre (53.0804, 31.0783) ccw
  line L147 (53.9242, 30.7537) -> (53.9242, 30.4292)
  arc A509 (53.9496, 30.7537) -> (53.8988, 30.7537) centre (53.9242, 30.7537) ccw
  line L148 (51.3842, 29.2749) -> (51.3842, 29.6644)
  arc A510 (53.5996, 31.1037) -> (53.5996, 31.0529) centre (53.5996, 31.0783) ccw
  line L149 (53.9242, 28.6399) -> (53.9242, 28.2504)
  arc A511 (52.7812, 28.6399) -> (52.7304, 28.6399) centre (52.7558, 28.6399) ccw
  arc A512 (53.9365, 29.8369) -> (53.9119, 29.8813) centre (53.9242, 29.8591) ccw
  arc A513 (53.9496, 28.6399) -> (53.8988, 28.6399) centre (53.9242, 28.6399) ccw
  arc A514 (52.7812, 28.2504) -> (52.7304, 28.2504) centre (52.7558, 28.2504) ccw
  arc A515 (53.9496, 28.2504) -> (53.8988, 28.2504) centre (53.9242, 28.2504) ccw
  arc A516 (37.4142, 29.5233) -> (36.7651, 29.5233) centre (37.0896, 29.5233) ccw
  arc A517 (36.2204, 29.5882) -> (36.2712, 29.5882) centre (36.2458, 29.5882) ccw
  arc A518 (53.8988, 28.2504) -> (53.9496, 28.2504) centre (53.9242, 28.2504) ccw
  arc A519 (36.7651, 29.5882) -> (36.2458, 29.5882) centre (36.5055, 29.5882) ccw
  arc A520 (36.7905, 29.5882) -> (36.7397, 29.5882) centre (36.7651, 29.5882) ccw
  arc A521 (53.9242, 28.6145) -> (53.9242, 28.6653) centre (53.9242, 28.6399) ccw
  line L150 (53.2751, 28.4452) -> (53.2751, 28.6399)
  arc A522 (53.2497, 28.4452) -> (53.3005, 28.4452) centre (53.2751, 28.4452) ccw
  arc A523 (53.6646, 27.9654) -> (53.6646, 28.0162) centre (53.6646, 27.9908) ccw
  arc A524 (37.0967, 28.0882) -> (37.1475, 28.0882) centre (37.1221, 28.0882) ccw
  line L151 (53.9242, 29.21) -> (52.7558, 29.21)
  line L152 (53.9242, 30.4292) -> (52.7558, 30.4292)
  line L153 (52.7558, 29.21) -> (53.9242, 29.8591)
  line L154 (53.9242, 29.8591) -> (52.7558, 29.8591)
  line L155 (53.2751, 28.6399) -> (53.9242, 28.6399)
  arc A525 (52.7558, 29.8845) -> (52.7558, 29.8337) centre (52.7558, 29.8591) ccw
  arc A526 (53.9242, 29.8337) -> (53.9242, 29.8845) centre (53.9242, 29.8591) ccw
  arc A527 (36.2712, 29.5882) -> (36.2204, 29.5882) centre (36.2458, 29.5882) ccw
  arc A528 (53.6646, 28.0162) -> (53.6646, 27.9654) centre (53.6646, 27.9908) ccw
  arc A529 (53.9242, 29.1846) -> (53.9242, 29.2354) centre (53.9242, 29.21) ccw
  line L156 (37.4142, 29.1987) -> (37.4142, 29.5233)
  arc A530 (36.7397, 29.5882) -> (36.7905, 29.5882) centre (36.7651, 29.5882) ccw
  arc A531 (36.7397, 29.5233) -> (36.7905, 29.5233) centre (36.7651, 29.5233) ccw
  line L157 (36.7651, 29.5882) -> (36.7651, 29.3285)
  line L158 (52.7558, 30.4292) -> (52.7558, 30.7537)
  arc A532 (52.7812, 30.7537) -> (52.7304, 30.7537) centre (52.7558, 30.7537) ccw
  arc A533 (36.2204, 29.1987) -> (36.2712, 29.1987) centre (36.2458, 29.1987) ccw
  line L159 (52.7558, 28.2504) -> (52.7558, 28.6399)
  arc A534 (52.7304, 30.4292) -> (52.7812, 30.4292) centre (52.7558, 30.4292) ccw
  line L160 (53.0804, 31.0783) -> (53.5996, 31.0783)
  arc A535 (53.6646, 27.9908) -> (53.9242, 28.2504) centre (53.6646, 28.2504) ccw
  arc A536 (53.2751, 28.6653) -> (53.2751, 28.6145) centre (53.2751, 28.6399) ccw
  arc A537 (52.7558, 30.4546) -> (52.7558, 30.4038) centre (52.7558, 30.4292) ccw
  line L161 (53.6646, 27.9908) -> (53.0154, 27.9908)
  arc A538 (51.3588, 29.2749) -> (51.4096, 29.2749) centre (51.3842, 29.2749) ccw
  line L162 (55.3085, 2.4892) -> (55.9576, 2.4892)
  arc A539 (59.4599, 1.2954) -> (59.4599, 1.3462) centre (59.4599, 1.3208) ccw
  arc A540 (58.1499, 1.5804) -> (58.0991, 1.5804) centre (58.1245, 1.5804) ccw
  line L163 (50.9298, 27.9908) -> (50.9298, 28.7697)
  arc A541 (57.3644, 1.8655) -> (57.3644, 1.8147) centre (57.3644, 1.8401) ccw
  arc A542 (59.4599, 1.3462) -> (59.4599, 1.2954) centre (59.4599, 1.3208) ccw
  arc A543 (58.0991, 1.5804) -> (58.1499, 1.5804) centre (58.1245, 1.5804) ccw
  arc A544 (61.5711, 2.4812) -> (61.5229, 2.4972) centre (61.547, 2.4892) ccw
  arc A545 (55.3085, 2.5146) -> (55.3085, 2.4638) centre (55.3085, 2.4892) ccw
  arc A546 (59.4599, 2.4638) -> (59.4599, 2.5146) centre (59.4599, 2.4892) ccw
  arc A547 (57.3644, 2.4638) -> (57.3644, 2.5146) centre (57.3644, 2.4892) ccw
  arc A548 (55.9576, 2.4638) -> (55.9576, 2.5146) centre (55.9576, 2.4892) ccw
  line L164 (61.1575, 1.3208) -> (61.547, 2.4892)
  arc A549 (59.1354, 2.5146) -> (59.1354, 2.4638) centre (59.1354, 2.4892) ccw
  line L165 (58.6438, 1.3208) -> (58.3842, 1.3208)
  line L166 (57.0399, 1.3208) -> (57.0399, 2.4892)
  arc A550 (58.3842, 1.3462) -> (58.3842, 1.2954) centre (58.3842, 1.3208) ccw
  line L167 (58.3842, 2.4892) -> (58.6438, 2.4892)
  arc A551 (59.1608, 2.4892) -> (59.11, 2.4892) centre (59.1354, 2.4892) ccw
  arc A552 (61.976, 1.3462) -> (61.976, 1.2954) centre (61.976, 1.3208) ccw
  arc A553 (59.4599, 1.9953) -> (59.4599, 1.9445) centre (59.4599, 1.9699) ccw
  line L168 (51.3193, 28.3803) -> (50.5404, 28.3803)
  arc A554 (50.5404, 28.4057) -> (50.5404, 28.3549) centre (50.5404, 28.3803) ccw
  arc A555 (59.4599, 1.9953) -> (59.4599, 1.9445) centre (59.4599, 1.9699) ccw
  arc A556 (61.1334, 1.3288) -> (61.1816, 1.3128) centre (61.1575, 1.3208) ccw
  arc A557 (57.3644, 1.8401) -> (57.3644, 2.4892) centre (57.3644, 2.1646) ccw
  arc A558 (58.6438, 2.4638) -> (58.6438, 2.5146) centre (58.6438, 2.4892) ccw
  arc A559 (62.3005, 1.3208) -> (62.3005, 1.9699) centre (62.3005, 1.6453) ccw
  line L169 (57.0399, 2.4892) -> (57.3644, 2.4892)
  line L170 (59.1354, 2.4892) -> (59.4599, 2.4892)
  arc A560 (62.3005, 1.2954) -> (62.3005, 1.3462) centre (62.3005, 1.3208) ccw
  line L171 (59.1354, 1.3208) -> (59.1354, 2.4892)
  line L172 (59.4599, 1.3208) -> (59.1354, 1.3208)
  arc A561 (59.1354, 1.3462) -> (59.1354, 1.2954) centre (59.1354, 1.3208) ccw
  arc A562 (59.11, 1.3208) -> (59.1608, 1.3208) centre (59.1354, 1.3208) ccw
  line L173 (58.1245, 1.5804) -> (58.1245, 2.2296)
  arc A563 (51.4096, 29.6644) -> (51.3588, 29.6644) centre (51.3842, 29.6644) ccw
  arc A564 (51.3842, 29.6644) -> (51.1246, 29.924) centre (51.1246, 29.6644) ccw
  arc A565 (59.4599, 2.5146) -> (59.4599, 2.4638) centre (59.4599, 2.4892) ccw
  arc A566 (50.9044, 27.9908) -> (50.9552, 27.9908) centre (50.9298, 27.9908) ccw
  arc A567 (58.0991, 2.2296) -> (58.1499, 2.2296) centre (58.1245, 2.2296) ccw
  arc A568 (58.1499, 2.2296) -> (58.0991, 2.2296) centre (58.1245, 2.2296) ccw
  arc A569 (57.0653, 2.4892) -> (57.0145, 2.4892) centre (57.0399, 2.4892) ccw
  arc A570 (60.7921, 2.4972) -> (60.7439, 2.4812) centre (60.768, 2.4892) ccw
  arc A571 (57.0145, 1.3208) -> (57.0653, 1.3208) centre (57.0399, 1.3208) ccw
  arc A572 (50.9552, 28.7697) -> (50.9044, 28.7697) centre (50.9298, 28.7697) ccw
  arc A573 (59.4599, 1.3208) -> (59.4599, 1.9699) centre (59.4599, 1.6453) ccw
  arc A574 (58.3842, 1.2954) -> (58.3842, 1.3462) centre (58.3842, 1.3208) ccw
  arc A575 (59.1354, 1.9953) -> (59.1354, 1.9445) centre (59.1354, 1.9699) ccw
  arc A576 (58.3842, 2.4892) -> (58.1245, 2.2296) centre (58.3842, 2.2295) ccw
  arc A577 (57.3644, 1.8147) -> (57.3644, 1.8655) centre (57.3644, 1.8401) ccw
  arc A578 (55.6076, 1.3208) -> (55.6584, 1.3208) centre (55.633, 1.3208) ccw
  arc A579 (51.3193, 28.3549) -> (51.3193, 28.4057) centre (51.3193, 28.3803) ccw
  arc A580 (58.3842, 2.4638) -> (58.3842, 2.5146) centre (58.3842, 2.4892) ccw
  arc A581 (59.4599, 1.9699) -> (59.4599, 2.4892) centre (59.4599, 2.2296) ccw
  arc A582 (51.3588, 29.6644) -> (51.4096, 29.6644) centre (51.3842, 29.6644) ccw
  arc A583 (59.4599, 1.9445) -> (59.4599, 1.9953) centre (59.4599, 1.9699) ccw
  line L174 (54.4288, 1.5804) -> (54.4288, 2.2296)
  arc A584 (53.4819, 2.5146) -> (53.4819, 2.4638) centre (53.4819, 2.4892) ccw
  line L175 (57.3644, 1.8401) -> (57.0399, 1.8401)
  line L176 (59.1354, 1.9699) -> (59.4599, 1.9699)
  line L177 (60.768, 2.4892) -> (61.1575, 1.3208)
  arc A585 (57.3644, 2.5146) -> (57.3644, 2.4638) centre (57.3644, 2.4892) ccw
  line L178 (6.3585, 1.1938) -> (6.7479, 2.3622)
  arc A586 (57.0399, 1.8655) -> (57.0399, 1.8147) centre (57.0399, 1.8401) ccw
  line L179 (5.969, 2.3622) -> (6.3585, 1.1938)
  arc A587 (13.9023, 1.1938) -> (13.9531, 1.1938) centre (13.9277, 1.1938) ccw
  arc A588 (12.9892, 1.1858) -> (13.0374, 1.2018) centre (13.0133, 1.1938) ccw
  arc A589 (14.0575, 1.1684) -> (14.0575, 1.2192) centre (14.0575, 1.1938) ccw
  line L180 (5.54, 1.4534) -> (5.54, 1.5833)
  line L181 (13.7978, 1.1938) -> (14.0575, 1.1938)
  arc A590 (62.3654, 1.9445) -> (62.3654, 1.9953) centre (62.3654, 1.9699) ccw
  arc A591 (4.8655, 1.8429) -> (4.9163, 1.8429) centre (4.8909, 1.8429) ccw
  arc A592 (13.4268, 2.3542) -> (13.3786, 2.3702) centre (13.4027, 2.3622) ccw
  line L182 (13.7978, 2.3622) -> (14.0575, 2.3622)
  arc A593 (57.0399, 2.5146) -> (57.0399, 2.4638) centre (57.0399, 2.4892) ccw
  arc A594 (14.0575, 2.3368) -> (14.0575, 2.3876) centre (14.0575, 2.3622) ccw
  line L183 (4.8909, 1.8429) -> (4.8909, 2.3622)
  arc A595 (5.2804, 1.8683) -> (5.2804, 1.8175) centre (5.2804, 1.8429) ccw
  arc A596 (5.5654, 1.4534) -> (5.5146, 1.4534) centre (5.54, 1.4534) ccw
  arc A597 (5.54, 2.3368) -> (5.54, 2.3876) centre (5.54, 2.3622) ccw
  line L184 (14.5556, 1.1938) -> (14.5556, 2.3622)
  arc A598 (4.8909, 1.2192) -> (4.8909, 1.1684) centre (4.8909, 1.1938) ccw
  arc A599 (14.581, 2.3622) -> (14.5302, 2.3622) centre (14.5556, 2.3622) ccw
  line L185 (61.976, 1.3208) -> (62.3005, 1.3208)
  arc A600 (5.5146, 1.5833) -> (5.5654, 1.5833) centre (5.54, 1.5833) ccw
  line L186 (4.8909, 2.3622) -> (5.54, 2.3622)
  arc A601 (5.2804, 1.8175) -> (5.2804, 1.8683) centre (5.2804, 1.8429) ccw
  arc A602 (62.1058, 1.9953) -> (62.1058, 1.9445) centre (62.1058, 1.9699) ccw
  line L187 (13.9277, 2.3622) -> (13.9277, 1.1938)
  arc A603 (62.3654, 1.9953) -> (62.3654, 1.9445) centre (62.3654, 1.9699) ccw
  arc A604 (61.976, 2.5146) -> (61.976, 2.4638) centre (61.976, 2.4892) ccw
  arc A605 (5.2804, 1.2192) -> (5.2804, 1.1684) centre (5.2804, 1.1938) ccw
  arc A606 (5.2804, 1.1938) -> (5.54, 1.4534) centre (5.2804, 1.4534) ccw
  line L188 (3.9963, 1.2587) -> (3.9963, 2.0376)
  arc A607 (3.6068, 1.6736) -> (3.6068, 1.6228) centre (3.6068, 1.6482) ccw
  arc A608 (58.6438, 1.2954) -> (58.6438, 1.3462) centre (58.6438, 1.3208) ccw
  arc A609 (4.8909, 1.8683) -> (4.8909, 1.8175) centre (4.8909, 1.8429) ccw
  arc A610 (6.3344, 1.1858) -> (6.3826, 1.2018) centre (6.3585, 1.1938) ccw
  arc A611 (13.7978, 1.2192) -> (13.7978, 1.1684) centre (13.7978, 1.1938) ccw
  arc A612 (5.54, 1.5833) -> (5.2804, 1.8429) centre (5.2804, 1.5833) ccw
  arc A613 (12.6479, 2.3702) -> (12.5997, 2.3542) centre (12.6238, 2.3622) ccw
  arc A614 (14.5778, 2.3745) -> (14.5334, 2.3499) centre (14.5556, 2.3622) ccw
  arc A615 (5.5146, 1.4534) -> (5.5654, 1.4534) centre (5.54, 1.4534) ccw
  line L189 (61.976, 2.4892) -> (62.3654, 2.4892)
  arc A616 (6.772, 2.3542) -> (6.7238, 2.3702) centre (6.7479, 2.3622) ccw
  arc A617 (5.2804, 1.1684) -> (5.2804, 1.2192) centre (5.2804, 1.1938) ccw
  line L190 (13.0133, 1.1938) -> (13.4027, 2.3622)
  arc A618 (61.1334, 1.3128) -> (61.1816, 1.3288) centre (61.1575, 1.3208) ccw
  arc A619 (4.0217, 2.0376) -> (3.9709, 2.0376) centre (3.9963, 2.0376) ccw
  arc A620 (4.9163, 2.3622) -> (4.8655, 2.3622) centre (4.8909, 2.3622) ccw
  arc A621 (4.3857, 1.6228) -> (4.3857, 1.6736) centre (4.3857, 1.6482) ccw
  arc A622 (5.5654, 1.5833) -> (5.5146, 1.5833) centre (5.54, 1.5833) ccw
  arc A623 (58.1245, 1.5804) -> (58.3842, 1.3208) centre (58.3842, 1.5805) ccw
  arc A624 (62.3005, 1.9953) -> (62.3005, 1.9445) centre (62.3005, 1.9699) ccw
  arc A625 (4.8909, 2.3876) -> (4.8909, 2.3368) centre (4.8909, 2.3622) ccw
  arc A626 (62.3654, 2.4638) -> (62.3654, 2.5146) centre (62.3654, 2.4892) ccw
  arc A627 (58.3842, 2.5146) -> (58.3842, 2.4638) centre (58.3842, 2.4892) ccw
  arc A628 (3.9709, 1.2587) -> (4.0217, 1.2587) centre (3.9963, 1.2587) ccw
  arc A629 (5.9931, 2.3702) -> (5.9449, 2.3542) centre (5.969, 2.3622) ccw
  line L191 (3.6068, 1.6482) -> (4.3857, 1.6482)
  arc A630 (6.3344, 1.2018) -> (6.3826, 1.1858) centre (6.3585, 1.1938) ccw
  arc A631 (62.3005, 1.3462) -> (62.3005, 1.2954) centre (62.3005, 1.3208) ccw
  arc A632 (62.3654, 1.9699) -> (62.3654, 2.4892) centre (62.3654, 2.2296) ccw
  line L192 (4.8909, 1.1938) -> (5.2804, 1.1938)
  arc A633 (12.9892, 1.2018) -> (13.0374, 1.1858) centre (13.0133, 1.1938) ccw
  line L193 (5.2804, 1.8429) -> (4.8909, 1.8429)
  arc A634 (40.3154, 19.1262) -> (40.3154, 19.0754) centre (40.3154, 19.1008) ccw
  arc A635 (41.2496, 19.7499) -> (41.1988, 19.7499) centre (41.2242, 19.7499) ccw
  arc A636 (22.7951, 20.3595) -> (22.7951, 20.4103) centre (22.7951, 20.3849) ccw
  arc A637 (15.1793, 1.1938) -> (15.2301, 1.1938) centre (15.2047, 1.1938) ccw
  arc A638 (13.7978, 2.3876) -> (13.7978, 2.3368) centre (13.7978, 2.3622) ccw
  line L194 (40.0558, 20.32) -> (41.2242, 20.9691)
  arc A639 (40.5497, 19.5552) -> (40.6005, 19.5552) centre (40.5751, 19.5552) ccw
  arc A640 (23.4696, 20.7744) -> (23.4188, 20.7744) centre (23.4442, 20.7744) ccw
  arc A641 (40.3154, 19.0754) -> (40.3154, 19.1262) centre (40.3154, 19.1008) ccw
  arc A642 (40.9646, 19.1008) -> (41.2242, 19.3604) centre (40.9646, 19.3604) ccw
  arc A643 (23.4362, 21.8284) -> (23.4522, 21.8766) centre (23.4442, 21.8525) ccw
  line L195 (41.2242, 20.9691) -> (40.0558, 20.9691)
  arc A644 (22.6004, 19.5157) -> (22.6004, 19.4649) centre (22.6004, 19.4903) ccw
  line L196 (22.7951, 20.3849) -> (22.2758, 20.3849)
  line L197 (22.9898, 19.1008) -> (22.9898, 19.8797)
  line L198 (14.5556, 2.3622) -> (15.2047, 1.1938)
  arc A645 (40.0558, 20.9945) -> (40.0558, 20.9437) centre (40.0558, 20.9691) ccw
  arc A646 (41.2242, 19.7245) -> (41.2242, 19.7753) centre (41.2242, 19.7499) ccw
  arc A647 (23.4188, 20.7744) -> (23.4696, 20.7744) centre (23.4442, 20.7744) ccw
  arc A648 (40.0558, 19.3604) -> (40.3154, 19.1008) centre (40.3154, 19.3604) ccw
  line L199 (23.1846, 21.034) -> (23.0547, 21.034)
  arc A649 (40.0812, 19.7499) -> (40.0304, 19.7499) centre (40.0558, 19.7499) ccw
  arc A650 (40.0304, 19.3604) -> (40.0812, 19.3604) centre (40.0558, 19.3604) ccw
  arc A651 (23.4188, 20.3849) -> (23.4696, 20.3849) centre (23.4442, 20.3849) ccw
  arc A652 (41.2496, 19.3604) -> (41.1988, 19.3604) centre (41.2242, 19.3604) ccw
  arc A653 (40.9646, 19.1262) -> (40.9646, 19.0754) centre (40.9646, 19.1008) ccw
  arc A654 (40.0812, 19.3604) -> (40.0304, 19.3604) centre (40.0558, 19.3604) ccw
  arc A655 (23.1846, 21.0086) -> (23.1846, 21.0594) centre (23.1846, 21.034) ccw
  arc A656 (22.2838, 22.266) -> (22.2678, 22.2178) centre (22.2758, 22.2419) ccw
  arc A657 (22.3012, 21.034) -> (22.2504, 21.034) centre (22.2758, 21.034) ccw
  arc A658 (40.9646, 19.0754) -> (40.9646, 19.1262) centre (40.9646, 19.1008) ccw
  line L200 (41.2242, 20.32) -> (40.0558, 20.32)
  arc A659 (22.8205, 20.7744) -> (22.7697, 20.7744) centre (22.7951, 20.7744) ccw
  arc A660 (22.2504, 20.3849) -> (22.3012, 20.3849) centre (22.2758, 20.3849) ccw
  arc A661 (22.2758, 20.4103) -> (22.2758, 20.3595) centre (22.2758, 20.3849) ccw
  arc A662 (23.1846, 21.0594) -> (23.1846, 21.0086) centre (23.1846, 21.034) ccw
  arc A663 (22.7697, 20.3849) -> (22.8205, 20.3849) centre (22.7951, 20.3849) ccw
  arc A664 (14.5302, 1.1938) -> (14.581, 1.1938) centre (14.5556, 1.1938) ccw
  arc A665 (62.3654, 2.5146) -> (62.3654, 2.4638) centre (62.3654, 2.4892) ccw
  line L201 (40.5751, 19.5552) -> (40.5751, 19.7499)
  arc A666 (15.2301, 2.3622) -> (15.1793, 2.3622) centre (15.2047, 2.3622) ccw
  arc A667 (22.9644, 19.1008) -> (23.0152, 19.1008) centre (22.9898, 19.1008) ccw
  arc A668 (23.4522, 21.8284) -> (23.4362, 21.8766) centre (23.4442, 21.8525) ccw
  arc A669 (40.5751, 19.7753) -> (40.5751, 19.7245) centre (40.5751, 19.7499) ccw
  line L202 (40.0558, 19.3604) -> (40.0558, 19.7499)
  line L203 (40.9646, 19.1008) -> (40.3154, 19.1008)
  line L204 (23.4442, 21.8525) -> (22.2758, 22.2419)
  arc A670 (22.7697, 20.7744) -> (22.8205, 20.7744) centre (22.7951, 20.7744) ccw
  arc A671 (40.6005, 19.7499) -> (40.5497, 19.7499) centre (40.5751, 19.7499) ccw
  line L205 (62.3654, 1.9699) -> (62.1058, 1.9699)
  arc A672 (23.0547, 21.0594) -> (23.0547, 21.0086) centre (23.0547, 21.034) ccw
  arc A673 (41.1988, 19.3604) -> (41.2496, 19.3604) centre (41.2242, 19.3604) ccw
  arc A674 (40.0435, 20.3422) -> (40.0681, 20.2978) centre (40.0558, 20.32) ccw
  line L206 (22.2758, 20.3849) -> (22.2758, 21.034)
  arc A675 (13.9531, 2.3622) -> (13.9023, 2.3622) centre (13.9277, 2.3622) ccw
  line L207 (23.3793, 19.4903) -> (22.6004, 19.4903)
  line L208 (23.4442, 20.3849) -> (23.4442, 20.7744)
  line L209 (12.6238, 2.3622) -> (13.0133, 1.1938)
  line L210 (15.2047, 1.1938) -> (15.2047, 2.3622)
  line L211 (41.2242, 19.7499) -> (41.2242, 19.3604)
  arc A676 (22.2678, 21.4871) -> (22.2838, 21.4389) centre (22.2758, 21.463) ccw
  arc A677 (15.1825, 1.1815) -> (15.2269, 1.2061) centre (15.2047, 1.1938) ccw
  arc A678 (23.4442, 20.7744) -> (23.1846, 21.034) centre (23.1846, 20.7744) ccw
  line L212 (22.2758, 21.463) -> (23.4442, 21.8525)
  arc A679 (41.1988, 52.5018) -> (41.2496, 52.5018) centre (41.2242, 52.5018) ccw
  line L213 (27.1893, 28.3803) -> (26.4104, 28.3803)
  line L214 (28.9504, 31.0783) -> (29.4696, 31.0783)
  arc A680 (24.8035, 54.4558) -> (24.8281, 54.4114) centre (24.8158, 54.4336) ccw
  arc A681 (24.8158, 55.1081) -> (24.8158, 55.0573) centre (24.8158, 55.0827) ccw
  arc A682 (27.2796, 29.6644) -> (27.2288, 29.6644) centre (27.2542, 29.6644) ccw
  line L215 (27.2542, 29.2749) -> (27.2542, 29.6644)
  arc A683 (27.2288, 29.2749) -> (27.2796, 29.2749) centre (27.2542, 29.2749) ccw
  arc A684 (27.2542, 29.6644) -> (26.9946, 29.924) centre (26.9946, 29.6644) ccw
  arc A685 (25.9842, 55.0573) -> (25.9842, 55.1081) centre (25.9842, 55.0827) ccw
  arc A686 (26.8252, 28.7697) -> (26.7744, 28.7697) centre (26.7998, 28.7697) ccw
  arc A687 (26.4104, 28.4057) -> (26.4104, 28.3549) centre (26.4104, 28.3803) ccw
  line L216 (26.9946, 29.924) -> (26.8647, 29.924)
  arc A688 (26.9946, 29.9494) -> (26.9946, 29.8986) centre (26.9946, 29.924) ccw
  line L217 (25.9842, 55.0827) -> (24.8158, 55.0827)
  line L218 (29.5346, 27.9908) -> (28.8854, 27.9908)
  arc A689 (26.0858, 29.3003) -> (26.0858, 29.2495) centre (26.0858, 29.2749) ccw
  arc A690 (40.2956, 53.667) -> (40.3353, 53.6988) centre (40.3154, 53.6829) ccw
  arc A691 (26.0938, 31.156) -> (26.0778, 31.1078) centre (26.0858, 31.1319) ccw
  arc A692 (29.5346, 28.0162) -> (29.5346, 27.9654) centre (29.5346, 27.9908) ccw
  line L219 (26.7998, 27.9908) -> (26.7998, 28.7697)
  arc A693 (27.1893, 28.3549) -> (27.1893, 28.4057) centre (27.1893, 28.3803) ccw
  arc A694 (26.7744, 27.9908) -> (26.8252, 27.9908) centre (26.7998, 27.9908) ccw
  arc A695 (27.2462, 30.7184) -> (27.2622, 30.7666) centre (27.2542, 30.7425) ccw
  arc A696 (27.2288, 29.6644) -> (27.2796, 29.6644) centre (27.2542, 29.6644) ccw
  arc A697 (25.9965, 55.0605) -> (25.9719, 55.1049) centre (25.9842, 55.0827) ccw
  arc A698 (40.0756, 54.0233) -> (40.036, 53.9916) centre (40.0558, 54.0075) ccw
  line L220 (33.6042, 53.6829) -> (33.6042, 54.332)
  arc A699 (41.2496, 52.8264) -> (41.1988, 52.8264) centre (41.2242, 52.8264) ccw
  arc A700 (29.1197, 28.4452) -> (29.1705, 28.4452) centre (29.1451, 28.4452) ccw
  line L221 (32.4358, 52.5018) -> (32.4358, 52.8264)
  line L222 (33.6042, 52.8264) -> (33.6042, 52.5018)
  arc A701 (33.6042, 55.1504) -> (32.9551, 55.1504) centre (33.2797, 55.1504) ccw
  arc A702 (32.9297, 55.1504) -> (32.9805, 55.1504) centre (32.9551, 55.1504) ccw
  arc A703 (40.2098, 54.8992) -> (40.2263, 54.9473) centre (40.2181, 54.9233) ccw
  line L223 (32.4358, 54.8259) -> (32.4358, 55.2154)
  line L224 (36.1442, 52.5018) -> (34.9758, 52.5018)
  arc A704 (32.4104, 55.2154) -> (32.4612, 55.2154) centre (32.4358, 55.2154) ccw
  arc A705 (36.1442, 52.4764) -> (36.1442, 52.5272) centre (36.1442, 52.5018) ccw
  arc A706 (40.0558, 54.0329) -> (40.0558, 53.9821) centre (40.0558, 54.0075) ccw
  arc A707 (33.2796, 53.1255) -> (33.2796, 53.1763) centre (33.2796, 53.1509) ccw
  arc A708 (32.7604, 53.1763) -> (32.7604, 53.1255) centre (32.7604, 53.1509) ccw
  arc A709 (33.2796, 53.1763) -> (33.2796, 53.1255) centre (33.2796, 53.1509) ccw
  arc A710 (33.5788, 52.8264) -> (33.6296, 52.8264) centre (33.6042, 52.8264) ccw
  arc A711 (32.4556, 54.0233) -> (32.416, 53.9916) centre (32.4358, 54.0075) ccw
  arc A712 (33.6296, 55.1504) -> (33.5788, 55.1504) centre (33.6042, 55.1504) ccw
  arc A713 (26.8647, 29.924) -> (26.6051, 29.6644) centre (26.8647, 29.6644) ccw
  arc A714 (32.4104, 52.5018) -> (32.4612, 52.5018) centre (32.4358, 52.5018) ccw
  arc A715 (40.0812, 55.1504) -> (40.0304, 55.1504) centre (40.0558, 55.1504) ccw
  arc A716 (32.4612, 52.8264) -> (32.4104, 52.8264) centre (32.4358, 52.8264) ccw
  line L225 (32.7604, 53.1509) -> (33.2796, 53.1509)
  line L226 (32.4358, 54.0075) -> (33.6042, 54.0075)
  line L227 (41.2242, 53.6829) -> (41.2242, 54.332)
  arc A717 (33.6296, 54.332) -> (33.5788, 54.332) centre (33.6042, 54.332) ccw
  arc A718 (32.4104, 54.8259) -> (32.4612, 54.8259) centre (32.4358, 54.8259) ccw
  arc A719 (40.2181, 55.3776) -> (40.0558, 55.1504) centre (40.296, 55.1504) ccw
  arc A720 (33.5788, 52.5018) -> (33.6296, 52.5018) centre (33.6042, 52.5018) ccw
  arc A721 (32.9551, 55.2154) -> (32.4358, 55.2154) centre (32.6955, 55.2154) ccw
  line L228 (33.6042, 54.8259) -> (33.6042, 55.1504)
  line L229 (40.3154, 53.6829) -> (40.0558, 54.0075)
  line L230 (40.0558, 54.0075) -> (41.2242, 54.0075)